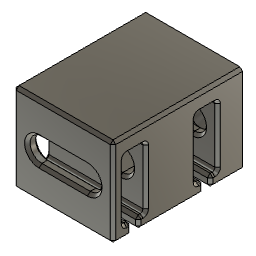
model (Autodesk Fusion 360 design; units mm, degrees)
Autodesk Fusion 360 part; units mm, degrees
sketch "Sketch1" plane through (0, 0, 0) normal (1, 0, 0) x (0, 1, 0)
  line L0 (-16.8, 22) -> (-9, 22)
  line L1 (-9, 22) -> (-9, 0)
  line L2 (-9, 0) -> (-16.8, 0)
  line L3 (-16.8, 0) -> (-16.8, 22)
  line L4 (-9, 0) -> (0, 0) construction
  line L5 (-14.1, 0) -> (-14.1, -4)
  line L6 (-11.7, 0) -> (-11.7, -4)
  line L7 (-14.1, -4) -> (-12.9, 0) construction
  line L8 (-11.7, -4) -> (-12.9, 0) construction
  line L9 (-14.1, -4) -> (-20.8, -4)
  line L10 (-20.8, -4) -> (-20.8, 28)
  line L11 (-20.8, 28) -> (0, 28)
  line L12 (0, 28) -> (0, -4)
  line L13 (0, -4) -> (-11.7, -4)
  line L14 (-6, 28) -> (-6, -4)
  line L15 (-9, 0) -> (-6, 0)
  line L16 (-20.8, 0) -> (-16.8, 0)
  line L17 (-16.8, 22) -> (-16.8, 28)
  line L18 (-16.8, 22) -> (-20.8, 22)
  dimension "d1" = 9
  dimension "d2" = 7.8
  dimension "d3" = 22
  dimension "d4" = 2.4
  dimension "d5" = 4
  dimension "d6" = 4
  dimension "d7" = 6
  dimension "d8" = 6
  constraint horizontal L0
  constraint vertical L1
  constraint horizontal L2
  constraint vertical L3
  constraint coincident L4.end origin
  constraint horizontal L4
  constraint coincident L2 L5.start
  constraint coincident L2 L6.start
  constraint vertical L5
  constraint vertical L6
  constraint equal L5 L6
  constraint midpoint L2 L7.end
  constraint equal L7 L8
  constraint horizontal L13
  constraint horizontal L9
  constraint vertical L10
  constraint horizontal L11
  constraint vertical L12
  constraint coincident L4.end L12
  constraint coincident L11 L14.start
  constraint coincident L13 L14.end
  constraint vertical L14
  constraint coincident L14 L15.end
  constraint coincident L4 L15.end
  constraint coincident L10 L16.start
  constraint perpendicular L3 L16
  constraint perpendicular L11 L17
  constraint coincident L10 L18.end
  constraint perpendicular L10 L18
  constraint coincident L11 L17.end
  measures "d1" horizontal distance of L4.end L1.end
  measures "d2" distance of L1.end L2.end
  measures "d3" distance of L0.start L2.end
  measures "d4" distance of L5.end L6.end
  measures "d5" vertical distance of L2.end L9.end
  measures "d6" horizontal distance of L2.end L9.end
  measures "d7" vertical distance of L0.start L10.end
  measures "d8" distance of L12.end L14.end
extrude "Extrude4" add sketch "Sketch1" along normal blind 36 contours L0 L1 L11 L14 L15 L17 | L10 L11 L17 L18 | L3 L10 L16 L18 | L2 L5 L9 L10 L16 | L2 L6 L13 L14 L15 | L11 L12 L13 L14 makes body 1
sketch "Sketch2" plane through (0, -20.8, 0) normal (0, -1, 0) x (1, 0, 0)
  line L0 (0, 28) -> (0, -4)
  line L1 (0, -4) -> (36, -4)
  line L2 (36, -4) -> (36, 28)
  line L3 (36, 28) -> (0, 28)
  circle A0 centre (9.25, 12) radius 2
  circle A1 centre (26.75, 12) radius 2
  line L4 (9.25, 12) -> (26.75, 12) construction
  line L5 (26.75, 12) -> (36, 12) construction
  line L6 (18, 12) -> (18, 28) construction
  circle A2 centre (9.25, 12) radius 4.25
  circle A3 centre (26.75, 12) radius 4.25
  line L7 (9.25, 16.25) -> (26.75, 16.25)
  line L8 (9.25, 7.75) -> (26.75, 7.75)
  point P0 (31, 12)
  dimension "d20" = 4
  dimension "d21" = 5
  dimension "d22" = 8.5
  constraint coincident A0.centre L4.start
  constraint coincident A1.centre L4.end
  constraint horizontal L4
  constraint midpoint L2 L5.end
  constraint horizontal L5
  constraint midpoint L4 L6.start
  constraint midpoint L3 L6.end
  constraint vertical L6
  constraint equal A0 A1
  constraint concentric A0 A2
  constraint concentric A1 A3
  constraint equal A2 A3
  constraint coincident A2 L7.start
  constraint coincident A3 L7.end
  constraint horizontal L7
  constraint coincident A2 L8.start
  constraint coincident A3 L8.end
  constraint parallel L4 L8
  constraint tangent A2 L8
  constraint tangent A2 L7
  constraint coincident L5 P0
  constraint coincident A3 P0
  measures "d20" diameter of A1
  measures "d21" distance of L5.end P0
  measures "d22" diameter of A3
copy_body "CopyPasteBodies1" bodies 1 makes body 2
move_body "Move1" bodies 2 to x (1, 0, 0) y (0, 1, 0) z (0, 0, 1) at (0, -26, 0)
extrude "Extrude7" add 1 faces at (24, -26, 17.3333) along direction (0, 1, 0) blind 6 on bodies 2 bodies 1 2
extrude "Extrude5" cut sketch "Sketch2" against normal up to surface (20.8 mm away) contours A0 | A1 bodies 1
extrude "Extrude6" cut sketch "Sketch2" along normal up to surface (-14.8 mm away) and the other way blind -38 contours A0 | A1 | A2 | A2 A3 L7 L8 | A3 bodies 1
chamfer "Chamfer3" distance 2.25 angle 45 2 edges at (7.3853, -6, 11.2768) (24.8853, -6, 11.2768) on bodies 1
fillet "Fillet2" radius 1 8 edges at (18, -9, 0) (18, -16.8, 0) (18, -42.8, 0) (18, -35, 0) (18, -35, 22) (18, -9, 22) (18, -16.8, 22) (18, -42.8, 22) on bodies 1
chamfer "Chamfer1" distance 1 angle 45 68 edges at (0, -16.8, 11) (0, -12.9, 22) (0, -9, 11) (0, -10.35, 0) (0, -15.45, 0) (36, -16.8, 11) (36, -12.9, 22) (36, -9, 11) (36, -10.35, 0) (36, -15.45, 0) (18, -9, 16.25) (31, -9, 12) (18, -9, 7.75) (5, -9, 12) (18, -16.8, 16.25) (5, -16.8, 12) (18, -16.8, 7.75) (31, -16.8, 12) (0, -11.7, -2) (0, -14.1, -2) (0, -5.85, -4) (0, -25.9, -4) (18, -11.7, -4) (18, -11.7, 0) (18, -14.1, -4) (0, -23.4, 28) (36, -23.4, 28) (36, -14.1, -2) (36, -11.7, -2) (36, -25.9, -4) (36, -5.85, -4) (18, -14.1, 0) (0, -46.8, 12) (18, -46.8, 28) (36, -46.8, 12) (18, -46.8, -4) (31, -42.8, 12) (18, -42.8, 16.25) (5, -42.8, 12) (18, -42.8, 7.75) (31, -46.8, 12) (18, -46.8, 7.75) (5, -46.8, 12) (18, -46.8, 16.25) (31, -35, 12) (18, -35, 7.75) (5, -35, 12) (18, -35, 16.25) (0, -35, 11) (0, -36.35, 0) (0, -37.7, -2) (18, -37.7, 0) (18, -40.1, 0) (0, -40.1, -2) (0, -41.45, 0) (0, -42.8, 11) (0, -38.9, 22) (0, -43.45, -4) (36, -38.9, 22) (36, -35, 11) (36, -42.8, 11) (36, -41.45, 0) (36, -36.35, 0) (36, -40.1, -2) (36, -37.7, -2) (18, -40.1, -4) (18, -37.7, -4) (36, -43.45, -4) on bodies 1
equation "d6 = d5"
equation "d7 = d8"
